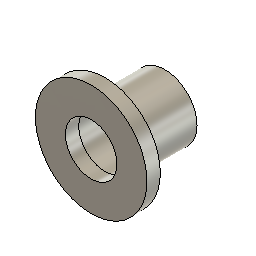
_Bushing.d676b754-ac8c-492a-baaf-132cd2dec664 (Autodesk Fusion 360 design; units mm, degrees)
Autodesk Fusion 360 part; units mm, degrees
sketch "Sketch1" plane through (0, 0, 0) normal (0, 0, 1) x (1, 0, 0)
  circle A0 centre (0, 0) radius 6
  circle A1 centre (0, 0) radius 2.85
  dimension "d1" = 12
  dimension "d2" = 5.7
  constraint coincident A0.centre A1.centre
  measures "d1" diameter of A0
  measures "d2" diameter of A1
extrude "Extrude1" add sketch "Sketch1" along normal blind 1.5 draft 2
sketch "Sketch2" plane through (0, 0, 0) normal (0, 0, -1) x (-1, 0, 0)
  circle A0 centre (0, 0) radius 2.85
  circle A1 centre (0, 0) radius 6
  circle A2 centre (0, 0) radius 3.5
  dimension "d5" = 7
  constraint concentric A0 A2
  measures "d5" diameter of A2
extrude "Extrude2" add sketch "Sketch2" along normal blind 6.5 contours A2
sketch "Sketch3" plane through (0, 0, -6.5) normal (0, 0, -1) x (-1, 0, 0)
  circle A0 centre (0, 0) radius 2.85
  circle A1 centre (0, 0) radius 3.5
  circle A2 centre (0, 0) radius 3.5
  circle A3 centre (0, 0) radius 1.5
  dimension "d8" = 3
  constraint coincident A0.centre A1.centre
  constraint concentric A2 A3
  measures "d8" diameter of A3
extrude "Extrude3" add sketch "Sketch3" against normal blind 2 contours A0
